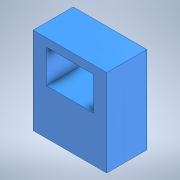
# Autodesk Inventor part: Pieza2
Saved by Autodesk Inventor 2021 (Build 250183000, 183)
## iProperties
Created: 2022-08-16
Part Number: Pieza2
Material: Genérico
Document SubType Name: Modeling
Designer: arthu
Density: 1 g/cm^3
Appearance: Cian
Author: arthu
Autodesk Inventor part; units mm, degrees
ref_plane "YZ Plane" through (0, 0, 0) normal (1, 0, 0) x (0, 1, 0)
ref_plane "XZ Plane" through (0, 0, 0) normal (0, 1, 0) x (-1, 0, 0)
ref_plane "XY Plane" through (0, 0, 0) normal (0, 0, 1) x (1, 0, 0)
sketch "Boceto1" plane through (0, 0, 0) normal (0, 0, 1) x (1, 0, 0)
  line L0 (17.5, -12.5) -> (-17.5, -12.5)
  line L1 (-17.5, -12.5) -> (-17.5, 12.5)
  line L2 (-17.5, 12.5) -> (17.5, 12.5)
  line L3 (17.5, 12.5) -> (17.5, -12.5)
  line L4 (17.5, -12.5) -> (-17.5, 12.5) construction
  line L5 (-17.5, -12.5) -> (17.5, 12.5) construction
  line L6 (-17.5, 12.5) -> (-7.5, 12.5) construction
  line L7 (-17.5, 12.5) -> (-27.5, 12.5)
  line L8 (-27.5, 12.5) -> (-27.5, 18.5)
  line L9 (-27.5, 18.5) -> (-17.5, 18.5)
  line L10 (-17.5, 18.5) -> (-17.5, 12.5)
  line L11 (-27.5, 18.5) -> (27.5, 18.5)
  line L12 (27.5, 18.5) -> (27.5, -46.5)
  line L13 (27.5, -46.5) -> (-27.5, -46.5)
  line L14 (-27.5, -46.5) -> (-27.5, 18.5)
  point P0 (0, 0)
  dimension "d0" = 35
  dimension "d1" = 25
  dimension "d4" = 10
  dimension "d5" = 6
  dimension "d6" = 55
  dimension "d7" = 65
  constraints: 30 end point, 6 parallel, 4 horizontal, 3 perpendicular, 2 midpoint
  measures "d0" distance of L1.end L2.end
  measures "d1" distance of L0.end L1.end
  measures "d4" distance of L8.end L9.end
  measures "d5" distance of L7.end L8.end
  measures "d6" distance of L12.end L13.end
  measures "d7" distance of L11.end L12.end
extrude "Extrusión1" add sketch "Boceto1" along normal blind 30
extrude "Extrusión2" add sketch "Boceto1" along normal blind 4 contours L0 L1 L2 L3
